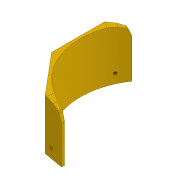
# Autodesk Inventor part: Delta Robot Siding Piece
Saved by Autodesk Inventor 2020 (Build 240168000, 168)
## iProperties
Created: 2021-04-12
Part Number: Delta Robot Siding Piece
Material: Generic
Document SubType Name: Modeling
Designer: Coy
Density: 1 g/cm^3
Appearance: Gold
Author: Coy
Autodesk Inventor part; units mm, degrees
ref_plane "YZ Plane" through (0, 0, 0) normal (1, 0, 0) x (0, 1, 0)
ref_plane "XZ Plane" through (0, 0, 0) normal (0, 1, 0) x (-1, 0, 0)
ref_plane "XY Plane" through (0, 0, 0) normal (0, 0, 1) x (1, 0, 0)
sketch "Sketch1" plane through (0, 0, 0) normal (0, 1, 0) x (-1, 0, 0)
  line L0 (68.675, -46.4884) -> (71.2969, -48.6885)
  line L1 (86.05, -31.1064) -> (71.2969, -48.6885)
  line L2 (86.05, 31.5329) -> (86.05, -31.1064)
  line L3 (45.7862, 79.5174) -> (86.05, 31.5329)
  line L4 (22.3355, 83.6524) -> (45.7862, 79.5174)
  line L5 (22.3355, 83.6524) -> (21.7555, 80.3631)
  arc A0 (68.675, -46.4884) -> (21.7555, 80.3631) centre (0, 0.2133) ccw
  constraints: 12 end point, 2 point on circle, 1 centre point
extrude "Extrusion1" add sketch "Sketch1" along normal blind 60
sketch "Sketch2" plane through (-86.05, 0, -31.1064) normal (-0.7660444, 0, -0.6427876) x (-0.6427876, 0, 0.7660444)
  circle A0 centre (-8.4518, 11) radius 1.625
  line L0 (-22.9518, 0) -> (0, 0) projected
  line L1 (-22.9518, 0) -> (-22.9518, 60) projected
  point P0 (-31.483, 0)
  dimension "d2" = 3.25
  dimension "d3" = 11
  dimension "d4" = 14.5
  constraints: 1 centre point
  measures "d2" diameter of A0
  measures "d3" distance from line of L0 A0.centre
  measures "d4" distance from line of L1 A0.centre
extrude "Extrusion2" cut sketch "Sketch2" against normal up to next
sketch "Sketch3" plane through (-22.3355, 0, 83.6524) normal (-0.1736482, 0, 0.9848078) x (0.9848078, 0, 0.1736482)
  circle A0 centre (-14.5, 11) radius 1.625
  line L0 (-23.8125, 0) -> (0, 0) projected
  line L1 (0, 0) -> (0, 60) projected
  point P0 (7.4701, 0)
  dimension "d7" = 3.25
  dimension "d8" = 11
  dimension "d9" = 14.5
  constraints: 1 centre point
  measures "d7" diameter of A0
  measures "d8" distance from line of L0 A0.centre
  measures "d9" distance from line of L1 A0.centre
extrude "Extrusion3" cut sketch "Sketch3" against normal up to next
chamfer "Chamfer5" distance 10 angle 45 2 edges at (-22.0455, 60, 82.0077) (-69.9859, 60, -47.5884)
chamfer "Chamfer6" distance 7 angle 45 2 edges at (-31.7611, 60, 79.5197) (-75.788, 60, -39.4028)
chamfer "Chamfer7" distance 5 angle 45 2 edges at (-38.4957, 60, 77.4021) (-79.5549, 60, -33.4258)
chamfer "Chamfer8" distance 5 angle 45 2 edges at (-22.0455, 50, 82.0077) (-69.9859, 50, -47.5884)
sketch "Sketch8" plane through (-86.05, 0, -31.1064) normal (-1, 0, 0) x (0, 0, 1)
  line L0 (0.07, 60.289) -> (62.7543, 60.289) construction
  line L1 (62.7543, 60.289) -> (62.7543, 0.051) construction
  line L2 (62.7543, 0.051) -> (0.07, 0.051) construction
  line L3 (0.07, 0.051) -> (0.07, 60.289) construction
  line L4 (4.1129, 46.045) -> (8.1352, 46.045)
  spline S0 degree 2 poles (8.1352, 46.045) (11.7291, 46.045) (14.4185, 44.8788) (15.799, 42.2369) (16.1322, 39.119) (16.1322, 34.7397) knots 0 0 0 1 2 3 4 4 4
  line L5 (16.1322, 34.7397) -> (16.1322, 23.9104)
  spline S1 degree 2 poles (16.1322, 23.9104) (16.1322, 19.6977) (15.6324, 16.7465) (14.3471, 14.9852) (12.4431, 14.295) (10.6342, 14.295) knots 0 0 0 1 2 3 4 4 4
  line L6 (10.6342, 14.295) -> (4.1129, 14.295)
  line L7 (4.1129, 14.295) -> (4.1129, 46.045)
  line L8 (9.7536, 39.952) -> (9.7536, 20.388)
  spline S2 degree 2 poles (9.7536, 20.388) (10.1106, 20.388) (10.4914, 21.4828) (10.4914, 24.5055) knots 0 0 0 1 2 2 2
  line L9 (10.4914, 24.5055) -> (10.4914, 36.5248)
  spline S3 degree 2 poles (10.4914, 36.5248) (10.4914, 38.5716) (10.3486, 39.595) (9.9916, 39.952) (9.7536, 39.952) knots 0 0 0 1 2 3 3 3
  line L10 (17.3936, 46.045) -> (26.2712, 46.045)
  line L11 (26.2712, 46.045) -> (26.2712, 39.0714)
  line L12 (26.2712, 39.0714) -> (23.0343, 39.0714)
  line L13 (23.0343, 39.0714) -> (23.0343, 34.0019)
  line L14 (23.0343, 34.0019) -> (26.057, 34.0019)
  line L15 (26.057, 34.0019) -> (26.057, 27.3139)
  line L16 (26.057, 27.3139) -> (23.0343, 27.3139)
  line L17 (23.0343, 27.3139) -> (23.0343, 21.2686)
  line L18 (23.0343, 21.2686) -> (26.5806, 21.2686)
  line L19 (26.5806, 21.2686) -> (26.5806, 14.295)
  line L20 (26.5806, 14.295) -> (17.3936, 14.295)
  line L21 (17.3936, 14.295) -> (17.3936, 46.045)
  line L22 (33.0306, 46.045) -> (33.0306, 21.2686)
  line L23 (33.0306, 21.2686) -> (35.9581, 21.2686)
  line L24 (35.9581, 21.2686) -> (35.9581, 14.295)
  line L25 (35.9581, 14.295) -> (27.3898, 14.295)
  line L26 (27.3898, 14.295) -> (27.3898, 46.045)
  line L27 (27.3898, 46.045) -> (33.0306, 46.045)
  line L28 (47.0729, 46.045) -> (47.0729, 39.0714)
  line L29 (47.0729, 39.0714) -> (44.2169, 39.0714)
  line L30 (44.2169, 39.0714) -> (44.2169, 14.295)
  line L31 (44.2169, 14.295) -> (38.5761, 14.295)
  line L32 (38.5761, 14.295) -> (38.5761, 39.0714)
  line L33 (38.5761, 39.0714) -> (35.7201, 39.0714)
  line L34 (35.7201, 39.0714) -> (35.7201, 46.045)
  line L35 (35.7201, 46.045) -> (47.0729, 46.045)
  line L36 (56.7122, 46.045) -> (59.5207, 14.295)
  line L37 (59.5207, 14.295) -> (53.8085, 14.295)
  line L38 (53.8085, 14.295) -> (53.5467, 19.8643)
  line L39 (53.5467, 19.8643) -> (52.5471, 19.8643)
  line L40 (52.5471, 19.8643) -> (52.2853, 14.295)
  line L41 (52.2853, 14.295) -> (46.5017, 14.295)
  line L42 (46.5017, 14.295) -> (48.977, 46.045)
  line L43 (48.977, 46.045) -> (56.7122, 46.045)
  spline S4 degree 2 poles (53.4039, 26.1477) (53.0469, 30.9792) (52.9517, 38.3574) knots 0 0 0 1 1 1
  spline S5 degree 2 poles (52.9517, 38.3574) (52.7375, 29.813) (52.5471, 26.1477) knots 0 0 0 1 1 1
  line L44 (52.5471, 26.1477) -> (53.4039, 26.1477)
  point P0 (31.1064, 0)
  constraints: 2 other
extrude "Extrusion8" add sketch "Sketch8" along normal blind 1.27
sketch "Sketch9" plane through (-45.7862, 0, 79.5174) normal (-0.7660444, 0, 0.6427876) x (0.6427876, 0, 0.7660444)
  line L0 (-62.4698, 60.3336) -> (-0.1509, 60.3336) construction
  line L1 (-0.1509, 60.3336) -> (-0.1509, -0.0863) construction
  line L2 (-0.1509, -0.0863) -> (-62.4698, -0.0863) construction
  line L3 (-62.4698, -0.0863) -> (-62.4698, 60.3336) construction
  line L4 (-13.3719, 11.0737) -> (-24.4252, 11.0737)
  line L5 (-24.4252, 11.0737) -> (-31.7735, 23.2076)
  line L6 (-31.7735, 23.2076) -> (-39.2762, 11.0737)
  line L7 (-39.2762, 11.0737) -> (-49.8664, 11.0737)
  line L8 (-49.8664, 11.0737) -> (-37.4854, 30.2472)
  line L9 (-37.4854, 30.2472) -> (-49.3724, 49.1737)
  line L10 (-49.3724, 49.1737) -> (-38.3191, 49.1737)
  line L11 (-38.3191, 49.1737) -> (-31.4339, 37.6572)
  line L12 (-31.4339, 37.6572) -> (-24.3635, 49.1737)
  line L13 (-24.3635, 49.1737) -> (-13.7733, 49.1737)
  line L14 (-13.7733, 49.1737) -> (-25.722, 30.6485)
  line L15 (-25.722, 30.6485) -> (-13.3719, 11.0737)
  point P0 (-31.483, 0)
  constraints: 2 other
extrude "Extrusion9" add sketch "Sketch9" along normal blind 1.27
body "Solid1"
